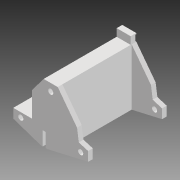
# Autodesk Inventor part: Knife Cart
Saved by Autodesk Inventor 2020 (Build 240168000, 168)
## iProperties
Created: 2020-10-19
Part Number: Knife Cart
Material: Generic
Document SubType Name: Modeling
Designer: DDeGo
Density: 1 g/cm^3
Appearance: Default
Author: DDeGo
Autodesk Inventor part; units mm, degrees
ref_plane "YZ Plane" through (0, 0, 0) normal (1, 0, 0) x (0, 1, 0)
ref_plane "XZ Plane" through (0, 0, 0) normal (0, 1, 0) x (-1, 0, 0)
ref_plane "XY Plane" through (0, 0, 0) normal (0, 0, 1) x (1, 0, 0)
sketch "Sketch2" plane through (0, 0, 0) normal (0, 0, 1) x (1, 0, 0)
  line L0 (-1.5, -7.5) -> (1.5, -7.5) construction
  line L1 (1.5, -7.5) -> (1.5, 7.5)
  line L2 (1.5, 7.5) -> (-1.5, 7.5)
  line L3 (-1.5, 7.5) -> (-1.5, -7.5)
  line L4 (-1.5, -7.5) -> (1.5, 7.5) construction
  line L5 (1.5, -7.5) -> (-1.5, 7.5) construction
  line L6 (-1.5, -7.5) -> (-3.5, -7.5)
  line L7 (1.5, -7.5) -> (3.5, -7.5)
  line L8 (3.5, -7.5) -> (47, 2.5)
  line L9 (47, 2.5) -> (47, 12.5)
  line L10 (47, 12.5) -> (35.1503, 28.1781) construction
  line L11 (14.5, 55.5) -> (-0.5, 55.5)
  line L12 (-0.5, 55.5) -> (-33, 12.5)
  line L13 (-33, 12.5) -> (-33, 2.5)
  line L14 (-33, 2.5) -> (-3.5, -7.5)
  line L15 (-33, 2.5) -> (47, 2.5) construction
  line L16 (47, 12.5) -> (-33, 12.5) construction
  line L17 (-33, 7.5) -> (47, 7.5) construction
  line L18 (7, 55.5) -> (7, 7.5) construction
  circle A0 centre (7, 47.5) radius 2.75
  circle A1 centre (-25, 7.5) radius 2.75
  circle A2 centre (39, 7.5) radius 2.75
  line L19 (-66.1508, 37.5) -> (80.1508, 37.5) construction
  line L20 (80.1508, 37.5) -> (80.1508, 17.5) construction
  line L21 (80.1508, 17.5) -> (-66.1508, 17.5) construction
  line L22 (-66.1508, 17.5) -> (-66.1508, 37.5) construction
  line L23 (-66.1508, 37.5) -> (80.1508, 17.5) construction
  line L24 (80.1508, 37.5) -> (-66.1508, 17.5) construction
  line L25 (35.1503, 28.1781) -> (37, 15.5)
  line L26 (37, 15.5) -> (47, 12.5)
  line L27 (35.1503, 28.1781) -> (14.5, 55.5)
  point P0 (0, 0)
  point P1 (7, 27.5)
  dimension "d6" = 10
  dimension "d7" = 3
  dimension "d8" = 15
  dimension "d10" = 2
  dimension "d11" = 40
  dimension "d12" = 8
  dimension "d13" = 5.5
  dimension "d14" = 8
  dimension "d15" = 8
  dimension "d16" = 80
  dimension "d17" = 15
  dimension "d18" = 20
  dimension "d19" = 20
  dimension "d20" = 10
  dimension "d31" = 25
  dimension "d40" = 10
  dimension "d41" = 3
  dimension "d42" = 115
  constraints: 56 end point, 8 midpoint, 6 parallel, 5 perpendicular, 4 horizontal, 4 point on line, 3 centre point, 2 collinear, 2 equal radius, 1 vertical
  measures "d6" distance between parallel lines of L16 L15
  measures "d7" distance of L1.end L2.end
  measures "d8" distance of L0.end L1.end
  measures "d10" distance of L0.start L6.end
  measures "d11" distance from line of A0.centre L17
  measures "d12" distance from line of L11 A0.centre
  measures "d13" diameter of A0
  measures "d14" distance from line of L13 A1.centre
  measures "d15" distance from line of L9 A2.centre
  measures "d16" distance of L9.end L12.end
  measures "d17" distance of L11.start L11.end
  measures "d18" distance of L19.end L20.end
  measures "d19" distance from line of L17 point (7, 27.5)
  measures "d20" distance between parallel lines of L21 L2
  measures "d31" horizontal distance of A1.centre point (0, 0)
  measures "d40" distance from line of L9 L25.end
  measures "d41" distance from line of L16 L25.end
  measures "d42" angle of L25 L26
extrude "Extrusion2" add sketch "Sketch2" along normal blind 84
sketch "Sketch3" plane through (-33, 2.5, 0) normal (-1, 0, 0) x (0, 0, 1)
  line L0 (0, 10) -> (0, 53) projected
  line L1 (0, 10) -> (25, 10)
  line L2 (25, 10) -> (25, 40)
  line L3 (25, 40) -> (0, 40)
  line L4 (0, 40) -> (0, 10)
  line L5 (84, 10) -> (84, 0) projected
  line L6 (84, 10) -> (59, 10)
  line L7 (59, 10) -> (59, 40)
  line L8 (59, 40) -> (84, 40)
  line L9 (84, 40) -> (84, 10)
  line L10 (25, 40) -> (59, 40) construction
  line L11 (0, 10) -> (84, 10) projected
  line L12 (29, -10) -> (55, -10)
  line L13 (55, -10) -> (55, 40)
  line L14 (55, 40) -> (29, 40)
  line L15 (29, 40) -> (29, -10)
  line L16 (0, -10) -> (84, -10) projected
  point P0 (0, -2.5)
  point P1 (55, 10)
  point P2 (29, 10)
  dimension "d23" = 30
  dimension "d24" = 25
  dimension "d32" = 4
  dimension "d33" = 4
  constraints: 26 end point, 6 parallel, 3 horizontal, 3 perpendicular, 3 point on line, 2 collinear
  measures "d23" distance of L1.end L2.end
  measures "d24" distance of L2.end L3.end
  measures "d32" distance between parallel lines of L2 L15
  measures "d33" distance between parallel lines of L7 L13
extrude "Extrusion3" cut sketch "Sketch3" against normal blind 20
sketch "Sketch4" plane through (47, 2.5, 0) normal (1, 0, 0) x (0, 0, -1)
  line L0 (-79, 53) -> (-5, 53)
  line L1 (-5, 53) -> (-5, -10)
  line L2 (-5, -10) -> (-79, -10)
  line L3 (-79, -10) -> (-79, 53)
  line L4 (0, 53) -> (-84, 53) projected
  line L5 (0, -10) -> (-84, -10) projected
  line L6 (-84, 0) -> (-84, 10) projected
  line L7 (0, 0) -> (0, 10) projected
  point P0 (0, -2.5)
  dimension "d43" = 5
  dimension "d44" = 5
  constraints: 8 end point, 2 parallel, 2 point on line, 1 horizontal, 1 perpendicular
  measures "d43" distance between parallel lines of L3 L6
  measures "d44" distance between parallel lines of L7 L1
extrude "Extrusion4" cut sketch "Sketch4" against normal blind 32.5
sketch "Sketch5" plane through (14.5, 2.5, 0) normal (1, 0, 0) x (0, 0, -1)
  line L0 (0, 53) -> (-84, 53) construction
  line L1 (0, 53) -> (-1, 53) construction
  line L2 (-6, 53) -> (-6, 61)
  line L3 (-6, 61) -> (0, 61)
  line L4 (0, 61) -> (0, 60)
  line L5 (0, 60) -> (-1, 60)
  line L6 (-1, 60) -> (-1, 53)
  line L7 (-1, 53) -> (-6, 53)
  line L8 (0, 60) -> (0, 53) construction
  point P0 (0, -2.5)
  dimension "d34" = 8
  dimension "d35" = 6
  dimension "d38" = 1
  dimension "d39" = 7
  constraints: 16 end point, 4 parallel, 3 horizontal, 3 perpendicular
  measures "d34" distance of L3.end L0.start
  measures "d35" distance of L2.end L3.end
  measures "d38" distance of L4.end L5.end
  measures "d39" distance of L5.end L1.end
extrude "Extrusion5" add sketch "Sketch5" against normal blind 15
equation "\"d14\" = d12"
equation "\"d15\" = d12"
body "Solid2"
